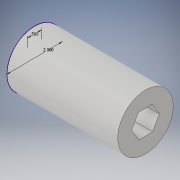
# Autodesk Inventor part: Roller
Saved by Autodesk Inventor 2017 (Build 210142000, 142)
## iProperties
Created: 2017-01-16
Part Number: Roller
Material: Generic
Document SubType Name: Modeling
Designer: mmarkle
Density: 1 g/cm^3
Appearance: Default
Author: mmarkle
Autodesk Inventor part; units mm, degrees
ref_plane "YZ Plane" through (0, 0, 0) normal (1, 0, 0) x (0, 1, 0)
ref_plane "XZ Plane" through (0, 0, 0) normal (0, 1, 0) x (-1, 0, 0)
ref_plane "XY Plane" through (0, 0, 0) normal (0, 0, 1) x (1, 0, 0)
sketch "Sketch1" plane through (0, 0, 0) normal (1, 0, 0) x (0, 1, 0)
  circle A0 centre (0, 0) radius 25.4
  line L0 (11.0708, -6.2248) -> (0.1446, -12.7)
  line L1 (0.1446, -12.7) -> (-10.9262, -6.4752)
  line L2 (-10.9262, -6.4752) -> (-11.0708, 6.2248)
  line L3 (-11.0708, 6.2248) -> (-0.1446, 12.7)
  line L4 (-0.1446, 12.7) -> (10.9262, 6.4752)
  line L5 (10.9262, 6.4752) -> (11.0708, -6.2248)
  dimension "d0" = 50.8
  dimension "d3" = 12.7
  constraints: 12 end point, 2 coincident, 1 centre point, 13 other
  measures "d0" diameter of A0
  measures "d3" vertical distance of L4.end L0.start
extrude "Extrusion1" add sketch "Sketch1" along normal blind 101.6 contours A0 | L0 L1 L2 L3 L4 L5
extrude "Extrusion2" cut sketch "Sketch1" along normal blind 101.6 contours L0 L1 L2 L3 L4 L5
body "Solid1"
